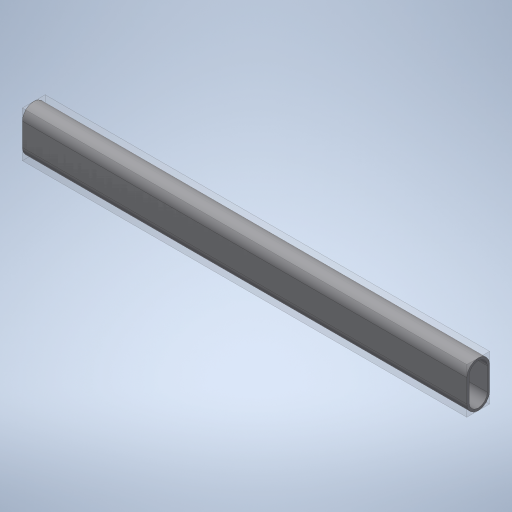
# Autodesk Inventor part: Oval Bar 30x15
Saved by Autodesk Inventor 2024 (Build 280153000, 153)
## iProperties
Created: 2015-03-09
Part Number: Oval Bar 30x15
Material: Generic
Description: Oval Wardrobe Bar
Document SubType Name: Modeling
Designer: SauliusD
Density: 1 g/cm^3
Appearance: Default
Bar_Length: 292.000 mm
Author: SauliusD
Autodesk Inventor part; units mm, degrees
ref_plane "YZ Plane" through (0, 0, 0) normal (1, 0, 0) x (0, 1, 0)
ref_plane "XZ Plane" through (0, 0, 0) normal (0, 1, 0) x (-1, 0, 0)
ref_plane "XY Plane" through (0, 0, 0) normal (0, 0, 1) x (1, 0, 0)
sketch "Sketch1" plane through (0, 0, 0) normal (0, 1, 0) x (-1, 0, 0)
  line L0 (-150, 15) -> (150, 15)
  line L1 (150, 15) -> (150, -15)
  line L2 (150, -15) -> (-150, -15)
  line L3 (-150, -15) -> (-150, 15)
  point P0 (0, -15)
  point P1 (0, 0)
  point P2 (150, 0)
  dimension "d1" = 30
  dimension "Length" = 300
  constraints: 8 end point, 2 midpoint, 2 parallel, 1 horizontal, 1 horizontal alignment, 1 perpendicular, 1 vertical alignment
  measures "d1" distance of L0.end L1.end
  measures "Length" distance of L0.start L0.end
sketch "Sketch2" plane through (0, 0, 0) normal (0, 1, 0) x (-1, 0, 0)
  line L0 (-150, 15) -> (150, 15) projected
  line L1 (150, -15) -> (-150, -15) projected
  line L2 (146, 15) -> (-146, 15)
  line L3 (-146, 15) -> (-146, -15)
  line L4 (-146, -15) -> (146, -15)
  line L5 (146, -15) -> (146, 15)
  point P0 (0, 0)
  dimension "d2" = 4
  dimension "d3" = 4
  dimension "Bar_Length" = 292
  constraints: 8 end point, 2 parallel, 2 point on line, 1 horizontal, 1 perpendicular
  measures "d2" distance from line of L0.end L5
  measures "d3" distance from line of L0.start L3
  measures "Bar_Length" distance between parallel lines of L3 L5
extrude "Extrusion1" add sketch "Sketch2" along normal mid plane 15
fillet "Fillet1" radius 7.5 4 edges at (0, -7.5, 15) (0, 7.5, 15) (0, -7.5, -15) (0, 7.5, -15)
shell "Shell1" thickness 1.5 removed faces 2 at (-146, 2.5, 2.5002) at (146, 2.5, -2.5002)
sketch "Sketch3" plane through (-146, 0, -7.5) normal (-1, 0, 0) x (0, 0, 1)
  line L0 (22.5, 7.5) -> (-7.5, 7.5)
  line L1 (-7.5, 7.5) -> (-7.5, -7.5)
  line L2 (-7.5, -7.5) -> (22.5, -7.5)
  line L3 (22.5, -7.5) -> (22.5, 7.5)
  arc A0 (15, -7.5) -> (15, 7.5) centre (15, 0) ccw projected
  arc A1 (0, 7.5) -> (0, -7.5) centre (0, 0) ccw projected
  line L4 (0, 7.5) -> (15, 7.5) projected
  line L5 (15, -7.5) -> (0, -7.5) projected
  point P0 (7.5, 0)
  constraints: 8 end point, 2 collinear, 2 parallel, 2 tangent, 1 horizontal, 1 perpendicular
extrude "Extrusion2" add sketch "Sketch3" against normal up to surface (292 mm away) separate body
equation "\"d6\" = 0.5 * d4"
equation "\"d4\" = 15"
body "Solid2"
